Autodesk Fusion 360 part; units mm, degrees
(part 2 of 7)
sketch "Sketch32" plane through (0, 0, 15.6) normal (0, 0, 1) x (-1, 0, 0)
  circle A0 centre (0, 19.7) radius 11.5
  circle A1 centre (-93.9, 19.7) radius 11.5
  line L0 (-126.4, -25.2) -> (-93.9, -25.2)
  line L1 (-93.9, -25.2) -> (-93.9, 4.1)
  line L2 (-93.9, 4.1) -> (0, 4.1)
  line L3 (0, 4.1) -> (0, -25.2)
  line L4 (0, -25.2) -> (32.5, -25.2)
  line L5 (32.5, -25.2) -> (32.5, 25.3)
  arc A2 (32.5, 25.3) -> (22.5, 35.3) centre (22.5, 25.3) ccw
  line L6 (22.5, 35.3) -> (-110.15, 35.3)
  line L7 (-110.15, 35.3) -> (-116.4, 35.3)
  arc A3 (-116.4, 35.3) -> (-126.4, 25.3) centre (-116.4, 25.3) ccw
  line L8 (-126.4, 25.3) -> (-126.4, -25.2)
  line L9 (-66.7, 10) -> (-66.7, 30.4)
  line L10 (-27.2, 30.4) -> (-27.2, 10)
  line L11 (-29.2, 8) -> (-64.7, 8)
  line L12 (-27.2, 30.4) -> (-34.2, 30.4)
  line L13 (-34.2, 30.4) -> (-34.2, 32.4)
  line L14 (-59.7, 32.4) -> (-59.7, 30.4)
  line L15 (-59.7, 30.4) -> (-66.7, 30.4)
  arc A4 (-66.7, 10) -> (-64.7, 8) centre (-64.7, 10) ccw
  arc A5 (-29.2, 8) -> (-27.2, 10) centre (-29.2, 10) ccw
  line L16 (-34.2, 30.4) -> (-34.2, 32.4)
  line L17 (-34.2, 32.4) -> (-59.7, 32.4)
  point P0 (-27.2, 4.5)
  point P1 (-66.7, 33.9)
  dimension "d199" = 3.5
  dimension "d205" = 2
  constraint vertical L9
  constraint vertical L10
  constraint perpendicular L9 L11
  constraint perpendicular L12 L13
  constraint perpendicular L9 L15
  constraint perpendicular L12 L16
  constraint perpendicular L14 L17
  measures "d199" distance of P1 L9.end
  measures "d205" distance of L12.end L13.end
extrude "Extrude23" cut sketch "Sketch32" against normal blind 1 contours L9 L10 L11 L12 L13 L14 L15 A4 A5 L16 L17 bodies 6 7
sketch "Sketch34" plane through (0, 0, 15.6) normal (0, 0, 1) x (-1, 0, 0)
  line L0 (-34.2, 32.4) -> (-34.2, 30.4)
  line L1 (-34.2, 30.4) -> (-27.2, 30.4)
  line L2 (-27.2, 30.4) -> (-27.2, 10)
  arc A0 (-29.2, 8) -> (-27.2, 10) centre (-29.2, 10) ccw
  line L3 (-29.2, 8) -> (-64.7, 8)
  arc A1 (-66.7, 10) -> (-64.7, 8) centre (-64.7, 10) ccw
  line L4 (-66.7, 10) -> (-66.7, 30.4)
  line L5 (-66.7, 30.4) -> (-59.7, 30.4)
  line L6 (-59.7, 30.4) -> (-59.7, 32.4)
  line L7 (-59.7, 32.4) -> (-34.2, 32.4)
  line L8 (-126.4, -25.2) -> (-93.9, -25.2)
  line L9 (-93.9, -25.2) -> (-93.9, 4.1)
  line L10 (-93.9, 4.1) -> (0, 4.1)
  line L11 (0, 4.1) -> (0, -25.2)
  line L12 (0, -25.2) -> (32.5, -25.2)
  line L13 (32.5, -25.2) -> (32.5, 25.3)
  arc A2 (32.5, 25.3) -> (22.5, 35.3) centre (22.5, 25.3) ccw
  line L14 (22.5, 35.3) -> (-110.15, 35.3)
  line L15 (-110.15, 35.3) -> (-116.4, 35.3)
  arc A3 (-116.4, 35.3) -> (-126.4, 25.3) centre (-116.4, 25.3) ccw
  line L16 (-126.4, 25.3) -> (-126.4, -25.2)
  line L17 (-46.95, 4.1) -> (-46.95, -15) construction
  circle A4 centre (0, 19.7) radius 11.5
  circle A5 centre (0, 19.7) radius 11.5
  line L18 (9, 20.7) -> (-9, 20.7)
  line L19 (0, 10.7) -> (5, 10.7)
  line L20 (5, 10.7) -> (-5, 10.7)
  arc A6 (5, 10.7) -> (4.9996, 12.7) centre (5, 11.7) ccw
  arc A7 (-4.9996, 12.7) -> (-5, 10.7) centre (-5, 11.7) ccw
  line L21 (0, 12.7) -> (5.0004, 12.7)
  line L22 (5.0004, 12.7) -> (-5.0004, 12.7)
  line L23 (8.1652, 14.7) -> (-8.1652, 14.7)
  line L24 (0, 14.7) -> (8.1652, 14.7)
  line L25 (0, 16.7) -> (8.1652, 16.7)
  line L26 (8.1652, 16.7) -> (-8.1652, 16.7)
  arc A8 (8.1652, 14.7) -> (8.1652, 16.7) centre (8.1652, 15.7) ccw
  arc A9 (-8.1652, 16.7) -> (-8.1652, 14.7) centre (-8.1652, 15.7) ccw
  arc A10 (-9, 20.7) -> (-9, 18.7) centre (-9, 19.7) ccw
  line L27 (-9, 18.7) -> (9, 18.7)
  arc A11 (9, 18.7) -> (9, 20.7) centre (9, 19.7) ccw
  line L28 (5, 28.7) -> (-5, 28.7)
  arc A12 (4.9996, 26.7) -> (5, 28.7) centre (5, 27.7) ccw
  line L29 (5.0004, 26.7) -> (-5.0004, 26.7)
  arc A13 (-5, 28.7) -> (-4.9996, 26.7) centre (-5, 27.7) ccw
  line L30 (8.1652, 24.7) -> (-8.1652, 24.7)
  arc A14 (-8.1652, 24.7) -> (-8.1652, 22.7) centre (-8.1652, 23.7) ccw
  arc A15 (8.1652, 22.7) -> (8.1652, 24.7) centre (8.1652, 23.7) ccw
  line L31 (8.1652, 22.7) -> (-8.1652, 22.7)
  arc A16 (-84.9, 18.7) -> (-84.9, 20.7) centre (-84.9, 19.7) ccw
  circle A17 centre (-93.9, 19.7) radius 11.5
  arc A18 (-102.9, 20.7) -> (-102.9, 18.7) centre (-102.9, 19.7) ccw
  circle A19 centre (-93.9, 19.7) radius 11.5
  line L32 (-102.0652, 14.7) -> (-85.7348, 14.7)
  line L33 (-93.9, 16.7) -> (-102.0652, 16.7)
  arc A20 (-102.0652, 24.7) -> (-102.0652, 22.7) centre (-102.0652, 23.7) ccw
  arc A21 (-88.9, 10.7) -> (-88.9004, 12.7) centre (-88.9, 11.7) ccw
  line L34 (-102.9, 20.7) -> (-84.9, 20.7)
  line L35 (-93.9, 14.7) -> (-102.0652, 14.7)
  line L36 (-102.0652, 24.7) -> (-85.7348, 24.7)
  arc A22 (-98.9, 28.7) -> (-98.8996, 26.7) centre (-98.9, 27.7) ccw
  line L37 (-98.9004, 12.7) -> (-88.8996, 12.7)
  line L38 (-93.9, 12.7) -> (-98.9004, 12.7)
  line L39 (-93.9, 10.7) -> (-98.9, 10.7)
  line L40 (-84.9, 18.7) -> (-102.9, 18.7)
  line L41 (-98.9, 28.7) -> (-88.9, 28.7)
  arc A23 (-98.8996, 12.7) -> (-98.9, 10.7) centre (-98.9, 11.7) ccw
  arc A24 (-88.9004, 26.7) -> (-88.9, 28.7) centre (-88.9, 27.7) ccw
  line L42 (-98.9004, 26.7) -> (-88.8996, 26.7)
  arc A25 (-85.7348, 14.7) -> (-85.7348, 16.7) centre (-85.7348, 15.7) ccw
  line L43 (-102.0652, 22.7) -> (-85.7348, 22.7)
  arc A26 (-102.0652, 16.7) -> (-102.0652, 14.7) centre (-102.0652, 15.7) ccw
  line L44 (-98.9, 10.7) -> (-88.9, 10.7)
  arc A27 (-85.7348, 22.7) -> (-85.7348, 24.7) centre (-85.7348, 23.7) ccw
  line L45 (-102.0652, 16.7) -> (-85.7348, 16.7)
  point P0 (-11.5, 19.7)
  point P1 (-82.4, 19.7)
  dimension "d328" = 2
  constraint midpoint L10 L17.start
  constraint perpendicular L10 L17
  constraint concentric A4 A5
  constraint coincident P0 A5
  constraint coincident A6.end L21
  constraint coincident A7 L22.end
  constraint coincident A6 L21.end
  constraint symmetric L17 A4 A17
  constraint symmetric L17 P0 P1
  constraint symmetric L17 A5 A19
  constraint symmetric L17 L25.start L33.start
  constraint symmetric L17 L24.start L35.start
  constraint symmetric L17 L21.start L38.start
  constraint symmetric L17 L19.start L39.start
  constraint symmetric L17 L19.end L39.end
  constraint symmetric L17 A6 A23
  constraint symmetric L17 A6.end A23.start
  constraint symmetric L17 L20.end A21.start
  constraint symmetric L17 A7.start A21.end
  constraint symmetric L17 A7 A21
  constraint symmetric L17 L22.end L37.end
  constraint symmetric L17 L21.end L37.start
  constraint symmetric L17 L25.end L33.end
  constraint symmetric L17 L23.start L32.start
  constraint symmetric L17 A8 A26
  constraint symmetric L17 L23.end L32.end
  constraint symmetric L17 A9 A25
  constraint symmetric L17 L26.end A25.end
  constraint symmetric L17 A10.end A16.start
  constraint symmetric L17 A10 A16
  constraint symmetric L17 L18.end A16.end
  constraint symmetric L17 L18.start A18.start
  constraint symmetric L17 L27.end A18.end
  constraint symmetric L17 A11 A18
  constraint symmetric L17 L28.start A22.start
  constraint symmetric L17 L28.end L41.end
  constraint symmetric L17 A12.start A22.end
  constraint symmetric L17 A12 A22
  constraint symmetric L17 L29.start L42.start
  constraint symmetric L17 L29.end L42.end
  constraint symmetric L17 A13.end A24.start
  constraint symmetric L17 A13 A24
  constraint symmetric L17 L30.start A20.start
  constraint symmetric L17 L30.end L36.end
  constraint symmetric L17 A14.end L43.end
  constraint symmetric L17 A14 A27
  constraint symmetric L17 A15.start A20.end
  constraint symmetric L17 A15 A20
  measures "d328" distance of L24.start L21.start
extrude "Extrude26" add sketch "Sketch34" against normal blind 1 contours A4 A5 | A17 A19 bodies 7
sketch "Sketch35" plane through (0, 0, 14.6) normal (0, 0, -1) x (1, 0, 0)
  line L0 (88.8996, 12.7) -> (98.8996, 12.7)
  arc A0 (98.9, 10.7) -> (98.8996, 12.7) centre (98.9, 11.7) ccw
  line L1 (98.9, 10.7) -> (88.9, 10.7)
  arc A1 (88.8996, 12.7) -> (88.9, 10.7) centre (88.9, 11.7) ccw
  line L2 (102.0652, 14.7) -> (85.7348, 14.7)
  arc A2 (85.7348, 16.7) -> (85.7348, 14.7) centre (85.7348, 15.7) ccw
  line L3 (85.7348, 16.7) -> (102.0652, 16.7)
  arc A3 (102.0652, 14.7) -> (102.0652, 16.7) centre (102.0652, 15.7) ccw
  arc A4 (102.0652, 22.7) -> (102.0652, 24.7) centre (102.0652, 23.7) ccw
  line L4 (102.0652, 22.7) -> (85.7348, 22.7)
  arc A5 (85.7348, 24.7) -> (85.7348, 22.7) centre (85.7348, 23.7) ccw
  line L5 (85.7348, 24.7) -> (102.0652, 24.7)
  arc A6 (98.9004, 26.7) -> (98.9, 28.7) centre (98.9, 27.7) ccw
  line L6 (98.9004, 26.7) -> (88.8996, 26.7)
  arc A7 (88.9, 28.7) -> (88.8996, 26.7) centre (88.9, 27.7) ccw
  line L7 (88.9, 28.7) -> (98.9, 28.7)
  arc A8 (102.9, 18.7) -> (102.9, 20.7) centre (102.9, 19.7) ccw
  line L8 (102.9, 18.7) -> (84.9, 18.7)
  arc A9 (84.9, 20.7) -> (84.9, 18.7) centre (84.9, 19.7) ccw
  line L9 (84.9, 20.7) -> (102.9, 20.7)
  line L10 (8.1652, 14.7) -> (-8.1652, 14.7)
  arc A10 (-8.1652, 16.7) -> (-8.1652, 14.7) centre (-8.1652, 15.7) ccw
  line L11 (-8.1652, 16.7) -> (8.1652, 16.7)
  arc A11 (8.1652, 14.7) -> (8.1652, 16.7) centre (8.1652, 15.7) ccw
  arc A12 (-9, 20.7) -> (-9, 18.7) centre (-9, 19.7) ccw
  line L12 (-9, 20.7) -> (9, 20.7)
  arc A13 (9, 18.7) -> (9, 20.7) centre (9, 19.7) ccw
  line L13 (9, 18.7) -> (-9, 18.7)
  line L14 (-8.1652, 24.7) -> (8.1652, 24.7)
  arc A14 (8.1652, 22.7) -> (8.1652, 24.7) centre (8.1652, 23.7) ccw
  line L15 (8.1652, 22.7) -> (-8.1652, 22.7)
  arc A15 (-8.1652, 24.7) -> (-8.1652, 22.7) centre (-8.1652, 23.7) ccw
  arc A16 (-5, 28.7) -> (-5.0004, 26.7) centre (-5, 27.7) ccw
  line L16 (-5, 28.7) -> (5, 28.7)
  arc A17 (4.9996, 26.7) -> (5, 28.7) centre (5, 27.7) ccw
  line L17 (4.9996, 26.7) -> (-5.0004, 26.7)
  arc A18 (-5.0004, 12.7) -> (-5, 10.7) centre (-5, 11.7) ccw
  line L18 (-5.0004, 12.7) -> (5.0004, 12.7)
  arc A19 (5, 10.7) -> (5.0004, 12.7) centre (5, 11.7) ccw
  line L19 (5, 10.7) -> (-5, 10.7)
  line L20 (34.2, 30.4) -> (34.2, 32.4)
  line L21 (34.2, 32.4) -> (59.7, 32.4)
  line L22 (59.7, 32.4) -> (59.7, 30.4)
  line L23 (59.7, 30.4) -> (66.7, 30.4)
  line L24 (66.7, 30.4) -> (66.7, 10)
  arc A20 (64.7, 8) -> (66.7, 10) centre (64.7, 10) ccw
  line L25 (64.7, 8) -> (29.2, 8)
  arc A21 (27.2, 10) -> (29.2, 8) centre (29.2, 10) ccw
  line L26 (27.2, 10) -> (27.2, 30.4)
  line L27 (27.2, 30.4) -> (34.2, 30.4)
  line L28 (93.9, -25.2) -> (126.4, -25.2)
  line L29 (126.4, -25.2) -> (126.4, 25.3)
  arc A22 (126.4, 25.3) -> (116.4, 35.3) centre (116.4, 25.3) ccw
  line L30 (116.4, 35.3) -> (110.15, 35.3)
  line L31 (110.15, 35.3) -> (-22.5, 35.3)
  arc A23 (-22.5, 35.3) -> (-32.5, 25.3) centre (-22.5, 25.3) ccw
  line L32 (-32.5, 25.3) -> (-32.5, -25.2)
  line L33 (-32.5, -25.2) -> (0, -25.2)
  line L34 (0, -25.2) -> (0, 4.1)
  line L35 (0, 4.1) -> (93.9, 4.1)
  line L36 (93.9, 4.1) -> (93.9, -25.2)
  circle A24 centre (0, 19.7) radius 11.5
  circle A25 centre (0, 19.7) radius 14
  line L37 (46.95, 4.1) -> (46.95, -7.4163) construction
  circle A26 centre (93.9, 19.7) radius 14
  circle A27 centre (93.9, 19.7) radius 11.5
  point P0 (0, 19.7)
  dimension "d335" = 28
  constraint coincident P0 A24.centre
  constraint midpoint L35 L37.start
  constraint perpendicular L35 L37
  constraint symmetric A24 L37 A27
  constraint symmetric A25 L37 A26
  measures "d335" diameter of A25
extrude "Extrude27" add sketch "Sketch35" along normal blind 1.5 contours A25 | A26 bodies 7
extrude "Extrude28" add 1 faces at (-10.2309, 68.7361, 13.1) along direction (0, 0, -1) blind 3.1 on bodies 5 bodies 5
sketch "Sketch36" plane through (0, 0, 10) normal (0, 0, -1) x (1, 0, 0)
  arc A0 (-32.5, -65.1) -> (-12.5, -85.1) centre (-12.5, -65.1) ccw
  line L0 (-12.5, -85.1) -> (106.4, -85.1)
  arc A1 (106.4, -85.1) -> (126.2303, -67.7) centre (106.4, -65.1) ccw
  line L1 (126.2303, -67.7) -> (93.9, -67.7)
  line L2 (93.9, -67.7) -> (93.9, -75.1)
  line L3 (93.9, -75.1) -> (0, -75.1)
  line L4 (0, -75.1) -> (0, -57.7)
  line L5 (0, -57.7) -> (-32.5, -57.7)
  line L6 (-32.5, -57.7) -> (-32.5, -65.1)
  line L7 (93.9, -75.1) -> (0, -75.1)
  line L8 (46.95, -75.1) -> (46.95, -85.1)
  line L9 (46.95, -80.1) -> (46.95, -77.15)
  circle A2 centre (46.95, -80.1) radius 2.95
  dimension "d340" = 2.95
  constraint coincident L2.end L3.start
  constraint coincident L3.end L4.start
  constraint midpoint L3 L8.start
  constraint midpoint L0 L8.end
  constraint midpoint L8 L9.start
  constraint perpendicular L0 L9
  constraint coincident L9.start A2.centre
  constraint coincident L9.end A2
  measures "d340" distance of L9.start L9.end
extrude "Extrude29" cut sketch "Sketch36" against normal blind 10 contours L8 L9 A2 | L8 L9 A2 bodies 5
sketch "Sketch37" plane through (0, 0, 15.6) normal (0, 0, 1) x (-1, 0, 0)
  circle A0 centre (-46.95, -80.1) radius 2.95
  arc A1 (12.5, -85.1) -> (32.5, -65.1) centre (12.5, -65.1) ccw
  line L0 (32.5, -65.1) -> (32.5, -57.7)
  line L1 (32.5, -57.7) -> (0, -57.7)
  line L2 (0, -57.7) -> (0, -75.1)
  line L3 (0, -75.1) -> (-93.9, -75.1)
  line L4 (-93.9, -75.1) -> (-93.9, -67.7)
  line L5 (-93.9, -67.7) -> (-126.2303, -67.7)
  arc A2 (-126.2303, -67.7) -> (-106.4, -85.1) centre (-106.4, -65.1) ccw
  line L6 (-106.4, -85.1) -> (12.5, -85.1)
  circle A3 centre (-46.95, -80.1) radius 2.95
  arc A4 (-47.45, -80.6) -> (-46.45, -80.6) centre (-46.95, -80.6) ccw
  arc A5 (-46.45, -79.6) -> (-47.45, -79.6) centre (-46.95, -79.6) ccw
  arc A6 (-45.65, -80.6) -> (-45.65, -79.6) centre (-45.65, -80.1) ccw
  line L7 (-45.65, -80.6) -> (-46.45, -80.6)
  line L8 (-47.45, -80.6) -> (-48.25, -80.6)
  line L9 (-48.25, -79.6) -> (-47.45, -79.6)
  line L10 (-46.45, -79.6) -> (-45.65, -79.6)
  arc A7 (-48.25, -79.6) -> (-48.25, -80.6) centre (-48.25, -80.1) ccw
  line L11 (-46.45, -80.6) -> (-47.45, -80.6)
  constraint concentric A0 A3
  constraint collinear L7 L8
  constraint collinear L9 L10
extrude "Extrude31" add sketch "Sketch37" against normal blind 1 contours A0 A3 bodies 5
sketch "Sketch39" plane through (0, 0, 14.6) normal (0, 0, -1) x (1, 0, 0)
  circle A0 centre (0, 19.7) radius 14
  line L0 (34.2, 30.4) -> (34.2, 32.4)
  line L1 (34.2, 32.4) -> (59.7, 32.4)
  line L2 (59.7, 32.4) -> (59.7, 30.4)
  line L3 (59.7, 30.4) -> (66.7, 30.4)
  line L4 (66.7, 30.4) -> (66.7, 10)
  arc A1 (64.7, 8) -> (66.7, 10) centre (64.7, 10) ccw
  line L5 (64.7, 8) -> (29.2, 8)
  arc A2 (27.2, 10) -> (29.2, 8) centre (29.2, 10) ccw
  line L6 (27.2, 10) -> (27.2, 30.4)
  line L7 (27.2, 30.4) -> (34.2, 30.4)
  line L8 (93.9, -25.2) -> (126.4, -25.2)
  line L9 (126.4, -25.2) -> (126.4, 25.3)
  arc A3 (126.4, 25.3) -> (116.4, 35.3) centre (116.4, 25.3) ccw
  line L10 (116.4, 35.3) -> (110.15, 35.3)
  line L11 (110.15, 35.3) -> (-22.5, 35.3)
  arc A4 (-22.5, 35.3) -> (-32.5, 25.3) centre (-22.5, 25.3) ccw
  line L12 (-32.5, 25.3) -> (-32.5, -25.2)
  line L13 (-32.5, -25.2) -> (0, -25.2)
  line L14 (0, -25.2) -> (0, 4.1)
  line L15 (0, 4.1) -> (93.9, 4.1)
  line L16 (93.9, 4.1) -> (93.9, -25.2)
  circle A5 centre (93.9, 19.7) radius 14
  line L17 (66.7, 4.5) -> (66.7, 4.1)
  line L18 (66.7, 4.1) -> (93.9, 4.1)
  line L19 (93.9, 4.1) -> (126.4, 4.1)
  line L20 (126.4, 4.1) -> (126.4, 25.3)
  line L21 (116.4, 35.3) -> (-22.5, 35.3)
  arc A6 (126.4, 25.3) -> (116.4, 35.3) centre (116.4, 25.3) ccw
  circle A7 centre (93.9, 19.7) radius 14
  line L22 (66.7, 4.5) -> (66.7, 33.9)
  line L23 (66.7, 33.9) -> (27.2, 33.9)
  line L24 (27.2, 33.9) -> (27.2, 4.1)
  line L25 (27.2, 4.1) -> (0, 4.1)
  line L26 (0, 4.1) -> (-32.5, 4.1)
  line L27 (-32.5, 4.1) -> (-32.5, 25.3)
  arc A8 (-22.5, 35.3) -> (-32.5, 25.3) centre (-22.5, 25.3) ccw
  circle A9 centre (0, 19.7) radius 14
  point P0 (66.7, 4.5)
  point P1 (79.9, 19.7)
  point P2 (66.7, 33.9)
  point P3 (27.2, 33.9)
  point P4 (-14, 19.7)
  constraint coincident P0 L17.start
  constraint coincident L15 L17.end
  constraint perpendicular L15 L17
  constraint coincident L15.end L16.start
  constraint coincident L9 L19.end
  constraint perpendicular L9 L19
  constraint coincident L9.end A3.start
  constraint coincident A3.end L10.start
  constraint coincident L11.end A4.start
  constraint concentric A5 A7
  constraint coincident A7 P1
  constraint coincident P2 L22.end
  constraint coincident P3 L23.end
  constraint coincident L15 L24.end
  constraint perpendicular L15 L24
  constraint coincident L14.end L15.start
  constraint coincident L12 L26.end
  constraint perpendicular L12 L26
  constraint coincident A4.end L12.start
  constraint coincident A4.end A8
  constraint concentric A0 A9
  constraint coincident A9 P4
extrude "Extrude32" add sketch "Sketch39" along normal blind 4.6 contours L4 L6 L9 A3 L10 L11 A4 L12 L15 L17 L18 L19 L20 L21 A6 L22 L23 L24 L25 L26 L27 A8 bodies 7
sketch "Sketch40" plane through (66.7, 0, 0) normal (-1, 0, 0) x (0, -1, 0)
  line L0 (30.4, 15.6) -> (10, 15.6)
  line L1 (10, 15.6) -> (10, 14.6)
  line L2 (10, 14.6) -> (4.1, 14.6)
  line L3 (4.1, 14.6) -> (4.1, 10)
  line L4 (4.1, 10) -> (33.9, 10)
  line L5 (33.9, 10) -> (33.9, 14.6)
  line L6 (33.9, 14.6) -> (30.4, 14.6)
  line L7 (30.4, 14.6) -> (30.4, 15.6)
  line L8 (4.1, 14.6) -> (8.7, 10)
  line L9 (4.1, 14.6) -> (10.6054, 14.6) construction
  line L10 (8.7, 10) -> (4.1, 10)
  line L11 (4.1, 14.6) -> (4.1, 10)
  dimension "d363" = 45
  constraint horizontal L9
  constraint coincident L2.end L3.start
  constraint coincident L4 L8.end
  constraint coincident L3.end L4.start
  measures "d363" angle of L8 L9
extrude "Extrude33" cut sketch "Sketch40" against normal blind 27.2 contours L3 L4 L8 L10 L11 bodies 7
sketch "Sketch42" plane through (27.2, 0, 0) normal (1, 0, 0) x (0, 1, 0)
  line L0 (-10, 15.6) -> (-30.4, 15.6)
  line L1 (-30.4, 15.6) -> (-30.4, 14.6)
  line L2 (-30.4, 14.6) -> (-33.9, 14.6)
  line L3 (-33.9, 14.6) -> (-33.9, 10)
  line L4 (-33.9, 10) -> (-4.1, 10)
  line L5 (-4.1, 10) -> (-4.1, 14.6)
  line L6 (-4.1, 14.6) -> (-10, 14.6)
  line L7 (-10, 14.6) -> (-10, 15.6)
  line L8 (-4.1, 14.6) -> (-8.7, 10)
  line L9 (-4.1, 14.6) -> (2.4054, 14.6) construction
  line L10 (-8.7, 10) -> (-4.1, 10)
  line L11 (-4.1, 10) -> (-4.1, 14.6)
  dimension "d369" = 135
  constraint horizontal L9
  constraint coincident L5.end L6.start
  constraint coincident L4 L8.end
  constraint coincident L4.end L5.start
  measures "d369" angle of L8 L9
extrude "Extrude35" cut sketch "Sketch42" against normal blind 27.2 contours L4 L5 L8 L10 L11 bodies 7
sketch "Sketch43" plane through (0, 0, 14.6) normal (0, 0, -1) x (1, 0, 0)
  line L0 (126.4, 4.1) -> (93.9, 4.1)
  line L1 (93.9, 4.1) -> (93.9, -25.2)
  line L2 (93.9, -25.2) -> (126.4, -25.2)
  line L3 (126.4, -25.2) -> (126.4, 4.1)
  line L4 (93.9, -25.2) -> (95.9, -25.2)
  line L5 (93.9, 4.1) -> (95.9, 4.1)
  line L6 (126.2303, -67.7) -> (93.9, -67.7)
  line L7 (93.9, -67.7) -> (95.9, -67.7)
  line L8 (95.9, -67.7) -> (95.9, 4.1)
  line L9 (93.9, 4.1) -> (93.9, -67.7)
  line L10 (0, -57.7) -> (-2, -57.7)
  line L11 (-32.5, 4.1) -> (0, 4.1)
  line L12 (0, 4.1) -> (-2, 4.1)
  line L13 (-2, -57.7) -> (-2, 4.1)
  line L14 (0, 4.1) -> (0, -57.7)
  point P0 (93.9, -67.7)
  point P1 (0, -57.7)
  point P2 (0, 4.1)
  dimension "d372" = 2
  dimension "d373" = 2
  dimension "d374" = 2
  dimension "d375" = 2
  dimension "d376" = 2
  constraint coincident L1.end L2.start
  constraint perpendicular L1 L4
  constraint coincident L0.end L1.start
  constraint perpendicular L1 L5
  constraint coincident P0 L6.end
  constraint parallel L6 L7
  constraint coincident P1 L10.start
  constraint perpendicular L9 L10
  constraint coincident P2 L11.end
  constraint parallel L11 L12
  measures "d372" distance of L1.end L4.end
  measures "d373" distance of L0.end L5.end
  measures "d374" distance of P0 L7.end
  measures "d375" distance of P1 L10.end
  measures "d376" distance of P2 L12.end
extrude "Extrude36" add sketch "Sketch43" along normal blind 4.6 contours L0 L1 L2 L4 L5 L8 L9 | L2 L4 L6 L7 L8 L9 | L10 L11 L12 L13 L14 bodies 3 4 5 7
sketch "Sketch44" plane through (0, 0, 10) normal (0, 0, -1) x (1, 0, 0)
  line L0 (-2, -57.7) -> (-32.5, -57.7)
  line L1 (-32.5, -57.7) -> (-32.5, -65.1)
  arc A0 (-32.5, -65.1) -> (-12.5, -85.1) centre (-12.5, -65.1) ccw
  line L2 (-12.5, -85.1) -> (106.4, -85.1)
  arc A1 (106.4, -85.1) -> (126.2303, -67.7) centre (106.4, -65.1) ccw
  line L3 (126.2303, -67.7) -> (95.9, -67.7)
  line L4 (95.9, -67.7) -> (95.9, 4.1)
  line L5 (95.9, 4.1) -> (126.4, 4.1)
  line L6 (126.4, 4.1) -> (126.4, 25.3)
  arc A2 (126.4, 25.3) -> (116.4, 35.3) centre (116.4, 25.3) ccw
  line L7 (116.4, 35.3) -> (-22.5, 35.3)
  arc A3 (-22.5, 35.3) -> (-32.5, 25.3) centre (-22.5, 25.3) ccw
  line L8 (-32.5, 25.3) -> (-32.5, 4.1)
  line L9 (-32.5, 4.1) -> (-2, 4.1)
  line L10 (-2, 4.1) -> (-2, -57.7)
  circle A4 centre (46.95, -80.1) radius 2.95
  line L11 (0, -75.1) -> (0, 5.7)
  arc A5 (8.6603, 8.7) -> (0, 5.7) centre (0, 19.7) ccw
  line L12 (8.6603, 8.7) -> (27.2, 8.7)
  line L13 (27.2, 8.7) -> (27.2, 33.9)
  line L14 (27.2, 33.9) -> (66.7, 33.9)
  line L15 (66.7, 33.9) -> (66.7, 8.7)
  line L16 (66.7, 8.7) -> (85.2397, 8.7)
  arc A6 (93.9, 5.7) -> (85.2397, 8.7) centre (93.9, 19.7) ccw
  line L17 (93.9, 5.7) -> (93.9, -75.1)
  line L18 (93.9, -75.1) -> (0, -75.1)
  line L19 (95.9, -67.7) -> (129, -67.7)
  line L20 (129, -67.7) -> (129, -88)
  line L21 (129, -88) -> (95.9, -88)
  line L22 (95.9, -88) -> (95.9, -67.7)
  line L23 (-2, -57.7) -> (-36.3118, -57.7)
  line L24 (-36.3118, -57.7) -> (-36.3118, -88)
  line L25 (-36.3118, -88) -> (-2, -88)
  line L26 (-2, -88) -> (-2, -57.7)
  constraint horizontal L19
  constraint vertical L20
  constraint horizontal L21
  constraint vertical L22
  constraint coincident L3.end L4.start
  constraint horizontal L23
  constraint vertical L24
  constraint horizontal L25
  constraint vertical L26
  constraint coincident L0.start L10.end
extrude "Extrude37" cut sketch "Sketch44" against normal blind 4.6 contours L0 L1 A0 L2 L23 L26 | L2 A1 L3 L19 L22 bodies 3
sketch "Sketch45" plane through (0, 0, 10) normal (0, 0, -1) x (1, 0, 0)
  line L0 (0, -75.1) -> (0, 5.7)
  arc A0 (8.6603, 8.7) -> (0, 5.7) centre (0, 19.7) ccw
  line L1 (8.6603, 8.7) -> (27.2, 8.7)
  line L2 (27.2, 8.7) -> (27.2, 33.9)
  line L3 (27.2, 33.9) -> (66.7, 33.9)
  line L4 (66.7, 33.9) -> (66.7, 8.7)
  line L5 (66.7, 8.7) -> (85.2397, 8.7)
  arc A1 (93.9, 5.7) -> (85.2397, 8.7) centre (93.9, 19.7) ccw
  line L6 (93.9, 5.7) -> (93.9, -75.1)
  line L7 (93.9, -75.1) -> (0, -75.1)
  circle A2 centre (46.95, -80.1) radius 2.95
  line L8 (95.9, -85.1) -> (95.9, 4.1)
  line L9 (95.9, 4.1) -> (126.4, 4.1)
  line L10 (126.4, 4.1) -> (126.4, 25.3)
  arc A3 (126.4, 25.3) -> (116.4, 35.3) centre (116.4, 25.3) ccw
  line L11 (116.4, 35.3) -> (-22.5, 35.3)
  arc A4 (-22.5, 35.3) -> (-32.5, 25.3) centre (-22.5, 25.3) ccw
  line L12 (-32.5, 25.3) -> (-32.5, 4.1)
  line L13 (-32.5, 4.1) -> (-2, 4.1)
  line L14 (-2, 4.1) -> (-2, -85.1)
  line L15 (-2, -85.1) -> (95.9, -85.1)
  line L16 (93.9, -75.1) -> (93.9, -77.2)
  line L17 (93.9, -77.2) -> (95.9, -77.2)
  line L18 (95.9, -77.2) -> (75.9, -77.2)
  line L19 (75.9, -77.2) -> (95.9, -77.2)
  line L20 (95.9, -77.2) -> (95.9, -85.1)
  line L21 (95.9, -85.1) -> (75.9, -85.1)
  line L22 (75.9, -85.1) -> (75.9, -77.2)
  dimension "d381" = 2.1
  dimension "d382" = 20
  constraint coincident L6.end L7.start
  constraint perpendicular L7 L16
  constraint coincident L8 L17.end
  constraint perpendicular L8 L17
  constraint perpendicular L8 L18
  constraint horizontal L19
  constraint vertical L20
  constraint horizontal L21
  constraint vertical L22
  constraint coincident L8.start L15.end
  measures "d381" distance of L6.end L16.end
  measures "d382" distance of L17.end L18.end
extrude "Extrude38" cut sketch "Sketch45" against normal blind 4.6 contours L8 L15 L17 L18 L19 L20 L21 L22 bodies 3
sketch "Sketch46" plane through (0, 0, 14.6) normal (0, 0, -1) x (1, 0, 0)
  line L0 (95.9, 4.1) -> (95.9, -77.2)
  line L1 (95.9, -77.2) -> (75.9, -77.2)
  line L2 (75.9, -77.2) -> (75.9, -85.1)
  line L3 (75.9, -85.1) -> (106.4, -85.1)
  arc A0 (106.4, -85.1) -> (126.4, -65.1) centre (106.4, -65.1) ccw
  line L4 (126.4, -65.1) -> (126.4, 4.1)
  line L5 (126.4, 4.1) -> (95.9, 4.1)
  line L6 (107.5299, -38.2671) -> (107.1448, -38.6523)
  line L7 (107.1448, -38.6523) -> (105.4477, -36.9552)
  line L8 (105.4477, -36.9552) -> (105.8329, -36.5701)
  arc A1 (107.9591, -29.4) -> (105.8329, -36.5701) centre (110.15, -33.95) ccw
  line L9 (107.9591, -29.4) -> (112.3409, -29.4)
  arc A2 (112.3409, -38.5) -> (112.3409, -29.4) centre (110.15, -33.95) ccw
  line L10 (112.3409, -38.5) -> (107.9591, -38.5)
  arc A3 (107.5299, -38.2671) -> (107.9591, -38.5) centre (110.15, -33.95) ccw
  line L11 (112.7701, -44.6329) -> (113.1552, -44.2477)
  line L12 (113.1552, -44.2477) -> (114.8523, -45.9448)
  line L13 (114.8523, -45.9448) -> (114.4671, -46.3299)
  arc A4 (112.3364, -53.5022) -> (114.4671, -46.3299) centre (110.15, -48.95) ccw
  line L14 (112.3364, -53.5022) -> (112.3364, -53.5)
  line L15 (112.3364, -53.5) -> (107.9591, -53.5)
  arc A5 (107.9591, -44.4) -> (107.9591, -53.5) centre (110.15, -48.95) ccw
  line L16 (107.9591, -44.4) -> (112.3409, -44.4)
  arc A6 (112.7701, -44.6329) -> (112.3409, -44.4) centre (110.15, -48.95) ccw
  line L17 (106.9671, -44.0701) -> (107.3523, -44.4552)
  line L18 (107.3523, -44.4552) -> (105.6552, -46.1523)
  line L19 (105.6552, -46.1523) -> (105.2701, -45.7671)
  arc A7 (98.115, -43.6717) -> (105.2701, -45.7671) centre (102.65, -41.45) ccw
  line L20 (98.115, -43.6717) -> (98.0852, -39.29)
  arc A8 (107.185, -39.2283) -> (98.0852, -39.29) centre (102.65, -41.45) ccw
  line L21 (107.185, -39.2283) -> (107.2148, -43.61)
  arc A9 (106.9671, -44.0701) -> (107.2148, -43.61) centre (102.65, -41.45) ccw
  line L22 (113.3329, -38.8299) -> (112.9477, -38.4448)
  line L23 (112.9477, -38.4448) -> (114.6448, -36.7477)
  line L24 (114.6448, -36.7477) -> (115.0299, -37.1329)
  arc A10 (122.2, -39.2591) -> (115.0299, -37.1329) centre (117.65, -41.45) ccw
  line L25 (122.2, -39.2591) -> (122.2, -43.6409)
  arc A11 (113.1, -43.6409) -> (122.2, -43.6409) centre (117.65, -41.45) ccw
  line L26 (113.1, -43.6409) -> (113.1, -39.2591)
  arc A12 (113.3329, -38.8299) -> (113.1, -39.2591) centre (117.65, -41.45) ccw
  circle A13 centre (102.6547, -56.4453) radius 2.85
  circle A14 centre (117.6453, -56.4453) radius 2.85
  line L27 (93.9, -75.1) -> (93.9, -62.1)
  line L28 (110.15, -48.95) -> (110.15, -75) construction
  line L29 (93.9, -62.1) -> (111.5, -62.1)
  line L30 (110.15, -62.1) -> (107.65, -62.1)
  circle A15 centre (110.15, -62.1) radius 2.5
  line L31 (126.4, -65.1) -> (-32.5, -65.1)
  line L32 (93.9, -62.1) -> (93.9, -65.1)
  line L33 (-2, -65.1) -> (-2, -62.1)
  line L34 (-2, -62.1) -> (-16.25, -62.1)
  circle A16 centre (-16.25, -62.1) radius 2.5
  line L35 (102.65, -41.45) -> (87.8982, -41.4191) construction
  circle A17 centre (110.2363, -20.8316) radius 2.5
  circle A18 centre (-16.1626, -20.3028) radius 2.5
  point P0 (93.9, -75.1)
  point P1 (-32.5, -65.1)
  dimension "d385" = 13
  dimension "d386" = 2.5
  dimension "d387" = 3
  dimension "d388" = 14.25
  dimension "d389" = 5
  constraint coincident P0 L27.start
  constraint parallel L0 L27
  constraint coincident A4.centre A5.centre
  constraint perpendicular L15 L28
  constraint perpendicular L28 L29
  constraint coincident L29 L30.start
  constraint coincident L28 L30.start
  constraint perpendicular L28 L30
  constraint coincident L30.start A15.centre
  constraint coincident L30.end A15
  constraint coincident A0.end L4.start
  constraint coincident P1 L31.end
  constraint coincident L27 L32.end
  constraint coincident L31 L32.end
  constraint coincident L31 L33.start
  constraint perpendicular L31 L33
  constraint perpendicular L33 L34
  constraint coincident L34.end A16.centre
  constraint coincident A7.centre A8.centre
  constraint symmetric A15 L35 A17
  constraint symmetric A16 L35 A18
  measures "d385" distance of P0 L27.end
  measures "d386" distance of L30.start L30.end
  measures "d387" distance of L33.start L33.end
  measures "d388" distance of L33.end L34.end
  measures "d389" diameter of A16
extrude "Extrude39" add sketch "Sketch46" along normal blind 1.6 contours A15 | A16 bodies 3
extrude "Extrude40" add sketch "Sketch46" along normal blind 1.6 contours A15 | A16 | A17 | A18 bodies 3
sketch "Sketch48" plane through (0, 0, 13) normal (0, 0, -1) x (1, 0, 0)
  circle A0 centre (110.15, -62.1) radius 2.5
  line L0 (110.15, -62.1) -> (109.75, -62.1)
  circle A1 centre (110.15, -62.1) radius 0.4
  circle A2 centre (110.2363, -20.8316) radius 0.4
  circle A3 centre (110.2363, -20.8316) radius 2.5
  circle A4 centre (-16.25, -62.1) radius 0.4
  circle A5 centre (-16.25, -62.1) radius 2.5
  circle A6 centre (-16.1626, -20.3028) radius 0.4
  circle A7 centre (-16.1626, -20.3028) radius 2.5
  dimension "d400" = 0.4
  dimension "d401" = 0.8
  dimension "d402" = 0.8
  dimension "d403" = 0.8
  constraint coincident A0.centre L0.start
  constraint horizontal L0
  constraint coincident L0.end A1
  constraint concentric A2 A3
  constraint concentric A4 A5
  constraint concentric A6 A7
  measures "d400" distance of A0.centre L0.end
  measures "d401" diameter of A2
  measures "d402" diameter of A4
  measures "d403" diameter of A6
extrude "Extrude42" cut sketch "Sketch48" against normal blind 0.5 contours A1 | A2 | A4 | A6 bodies 3
sketch "Sketch49" plane through (0, 0, 10) normal (0, 0, -1) x (1, 0, 0)
  line L0 (75.9, -77.2) -> (95.9, -77.2)
  line L1 (95.9, -77.2) -> (95.9, 4.1)
  line L2 (95.9, 4.1) -> (126.4, 4.1)
  line L3 (126.4, 4.1) -> (126.4, 25.3)
  arc A0 (126.4, 25.3) -> (116.4, 35.3) centre (116.4, 25.3) ccw
  line L4 (116.4, 35.3) -> (-22.5, 35.3)
  arc A1 (-22.5, 35.3) -> (-32.5, 25.3) centre (-22.5, 25.3) ccw
  line L5 (-32.5, 25.3) -> (-32.5, 4.1)
  line L6 (-32.5, 4.1) -> (-2, 4.1)
  line L7 (-2, 4.1) -> (-2, -85.1)
  line L8 (-2, -85.1) -> (75.9, -85.1)
  line L9 (75.9, -85.1) -> (75.9, -77.2)
  line L10 (0, -75.1) -> (0, 5.7)
  arc A2 (8.6603, 8.7) -> (0, 5.7) centre (0, 19.7) ccw
  line L11 (8.6603, 8.7) -> (27.2, 8.7)
  line L12 (27.2, 8.7) -> (27.2, 33.9)
  line L13 (27.2, 33.9) -> (66.7, 33.9)
  line L14 (66.7, 33.9) -> (66.7, 8.7)
  line L15 (66.7, 8.7) -> (85.2397, 8.7)
  arc A3 (93.9, 5.7) -> (85.2397, 8.7) centre (93.9, 19.7) ccw
  line L16 (93.9, 5.7) -> (93.9, -75.1)
  line L17 (93.9, -75.1) -> (0, -75.1)
  circle A4 centre (46.95, -80.1) radius 2.95
  line L18 (95.9, -77.2) -> (-2, -77.2)
  line L19 (-2, -77.2) -> (-2, 4.1)
  line L20 (-2, 4.1) -> (95.9, 4.1)
  line L21 (95.9, 4.1) -> (95.9, -77.2)
  line L22 (93.9, -75.1) -> (0, -75.1)
  line L23 (0, -75.1) -> (0, 4.1)
  line L24 (0, 4.1) -> (93.9, 4.1)
  line L25 (93.9, 4.1) -> (93.9, -75.1)
  point P0 (0, 4.1)
  constraint horizontal L18
  constraint vertical L19
  constraint horizontal L20
  constraint vertical L21
  constraint coincident L6.end L7.start
  constraint coincident L0.end L1.start
  constraint horizontal L22
  constraint vertical L23
  constraint horizontal L24
  constraint vertical L25
  constraint coincident P0 L23.end
  constraint coincident L16.end L17.start
extrude "Extrude43" add sketch "Sketch49" along normal blind 6 contours L0 L1 L7 L10 L16 L17 A4 L18 L19 L20 L21 L22 L23 L25 bodies 3
sketch "Sketch52" plane through (0, 0, 14.6) normal (0, 0, -1) x (1, 0, 0)
  circle A0 centre (110.2363, -20.8316) radius 2.5
  circle A1 centre (110.15, -62.1) radius 2.5
  line L0 (95.9, 4.1) -> (95.9, -77.2)
  line L1 (95.9, -77.2) -> (75.9, -77.2)
  line L2 (75.9, -77.2) -> (75.9, -85.1)
  line L3 (75.9, -85.1) -> (106.4, -85.1)
  arc A2 (106.4, -85.1) -> (126.4, -65.1) centre (106.4, -65.1) ccw
  line L4 (126.4, -65.1) -> (126.4, 4.1)
  line L5 (126.4, 4.1) -> (95.9, 4.1)
  line L6 (107.5299, -38.2671) -> (107.1448, -38.6523)
  line L7 (107.1448, -38.6523) -> (105.4477, -36.9552)
  line L8 (105.4477, -36.9552) -> (105.8329, -36.5701)
  arc A3 (107.9591, -29.4) -> (105.8329, -36.5701) centre (110.15, -33.95) ccw
  line L9 (107.9591, -29.4) -> (112.3409, -29.4)
  arc A4 (112.3409, -38.5) -> (112.3409, -29.4) centre (110.15, -33.95) ccw
  line L10 (112.3409, -38.5) -> (107.9591, -38.5)
  arc A5 (107.5299, -38.2671) -> (107.9591, -38.5) centre (110.15, -33.95) ccw
  line L11 (112.7701, -44.6329) -> (113.1552, -44.2477)
  line L12 (113.1552, -44.2477) -> (114.8523, -45.9448)
  line L13 (114.8523, -45.9448) -> (114.4671, -46.3299)
  arc A6 (112.3364, -53.5022) -> (114.4671, -46.3299) centre (110.15, -48.95) ccw
  line L14 (112.3364, -53.5022) -> (112.3364, -53.5)
  line L15 (112.3364, -53.5) -> (107.9591, -53.5)
  arc A7 (107.9591, -44.4) -> (107.9591, -53.5) centre (110.15, -48.95) ccw
  line L16 (107.9591, -44.4) -> (112.3409, -44.4)
  arc A8 (112.7701, -44.6329) -> (112.3409, -44.4) centre (110.15, -48.95) ccw
  line L17 (106.9671, -44.0701) -> (107.3523, -44.4552)
  line L18 (107.3523, -44.4552) -> (105.6552, -46.1523)
  line L19 (105.6552, -46.1523) -> (105.2701, -45.7671)
  arc A9 (98.115, -43.6717) -> (105.2701, -45.7671) centre (102.65, -41.45) ccw
  line L20 (98.115, -43.6717) -> (98.0852, -39.29)
  arc A10 (107.185, -39.2283) -> (98.0852, -39.29) centre (102.65, -41.45) ccw
  line L21 (107.185, -39.2283) -> (107.2148, -43.61)
  arc A11 (106.9671, -44.0701) -> (107.2148, -43.61) centre (102.65, -41.45) ccw
  line L22 (113.3329, -38.8299) -> (112.9477, -38.4448)
  line L23 (112.9477, -38.4448) -> (114.6448, -36.7477)
  line L24 (114.6448, -36.7477) -> (115.0299, -37.1329)
  arc A12 (122.2, -39.2591) -> (115.0299, -37.1329) centre (117.65, -41.45) ccw
  line L25 (122.2, -39.2591) -> (122.2, -43.6409)
  arc A13 (113.1, -43.6409) -> (122.2, -43.6409) centre (117.65, -41.45) ccw
  line L26 (113.1, -43.6409) -> (113.1, -39.2591)
  arc A14 (113.3329, -38.8299) -> (113.1, -39.2591) centre (117.65, -41.45) ccw
  circle A15 centre (102.6547, -56.4453) radius 2.85
  circle A16 centre (117.6453, -56.4453) radius 2.85
  line L27 (95.9, 4.1) -> (95.9, -0.9)
  line L28 (95.9, -0.9) -> (98.4, -0.9)
  line L29 (95.9, 4.1) -> (98.4, 4.1)
  line L30 (100.9, 1.6) -> (100.9, 4.1)
  line L31 (100.9, 4.1) -> (95.9, 4.1)
  circle A17 centre (98.4, 1.6) radius 0.4
  line L32 (93.9, -75.1) -> (0, -75.1)
  line L33 (46.95, -75.1) -> (46.95, -46.628) construction
  circle A18 centre (-4.5, 1.6) radius 0.4
  line L34 (-2, -0.9) -> (-4.5, -0.9)
  line L35 (-7, 1.6) -> (-7, 4.1)
  line L36 (-2, 4.1) -> (-4.5, 4.1)
  line L37 (-2, 4.1) -> (-2, 1.6)
  arc A19 (-7, 1.6) -> (-4.5, -0.9) centre (-4.5, 1.6) ccw
  arc A20 (98.4, -0.9) -> (100.9, 1.6) centre (98.4, 1.6) ccw
  line L38 (-2, 1.6) -> (-2, -0.9)
  line L39 (-7, 4.1) -> (-4.5, 4.1)
  line L40 (100.9, 4.1) -> (98.4, 4.1)
  line L41 (95.9, -0.9) -> (95.9, 4.1)
  line L42 (95.9, -0.9) -> (98.4, -0.9)
  dimension "d412" = 5
  dimension "d414" = 0.8
  constraint coincident L0.start L5.end
  constraint perpendicular L5 L27
  constraint tangent L28 A20
  constraint tangent L29 A20
  constraint coincident L5 L30.end
  constraint tangent L30 A20
  constraint perpendicular L5 L30
  constraint concentric A17 A20
  constraint midpoint L32 L33.start
  constraint perpendicular L32 L33
  constraint symmetric L0.start L33 L36.start
  constraint symmetric L27.end L33 L34.start
  constraint symmetric L30.start L33 L35.start
  constraint symmetric L33 A19 A20
  constraint symmetric L28.end L33 L34.end
  constraint symmetric L29.end L33 L36.end
  constraint symmetric L30.end L33 L35.end
  constraint symmetric A17 L33 A18
  constraint perpendicular L34 L38
  measures "d412" distance of L0.start L27.end
  measures "d414" diameter of A17
extrude "Extrude45" add sketch "Sketch52" along normal blind 10.6 contours L0 L5 L27 L28 L29 L30 L31 A20 L40 L41 L42 | L34 L35 L36 L37 A19 L38 L39 bodies 3
sketch "Sketch53" plane through (0, 0, 10) normal (0, 0, -1) x (1, 0, 0)
  line L0 (46.4092, -77.2) -> (-2, -77.2)
  line L1 (-2, -77.2) -> (-2, -85.1)
  line L2 (-2, -85.1) -> (75.9, -85.1)
  line L3 (75.9, -85.1) -> (75.9, -77.2)
  line L4 (75.9, -77.2) -> (47.4908, -77.2)
  arc A0 (46.4092, -77.2) -> (47.4908, -77.2) centre (46.95, -80.1) ccw
  line L5 (-2, -81.15) -> (18, -81.15)
  circle A1 centre (8, -81.15) radius 2.5
  circle A2 centre (8, -81.15) radius 0.4
  line L6 (10.5, -81.15) -> (10.5, -77.2)
  line L7 (5.5, -81.15) -> (5.5, -77.2)
  line L8 (5.5, -77.2) -> (10.5, -77.2)
  line L9 (8, -81.15) -> (75.9, -81.15)
  line L10 (75.9, -81.15) -> (70.9, -81.15)
  circle A3 centre (73.4, -81.15) radius 2.5
  line L11 (70.9, -81.15) -> (70.9, -77.2)
  line L12 (75.9, -81.15) -> (75.9, -77.2)
  line L13 (75.9, -77.2) -> (70.9, -77.2)
  circle A4 centre (73.4, -81.15) radius 0.4
  dimension "d420" = 20
  dimension "d421" = 5
  dimension "d422" = 0.8
  dimension "d440" = 5
  dimension "d441" = 0.8
  constraint midpoint L1 L5.start
  constraint perpendicular L1 L5
  constraint midpoint L5 A1.centre
  constraint concentric A1 A2
  constraint coincident A1 L6.start
  constraint coincident L5 L6.start
  constraint coincident L0 L6.end
  constraint tangent A1 L6
  constraint coincident A1 L7.start
  constraint coincident L5 L7.start
  constraint coincident L0 L7.end
  constraint tangent A1 L7
  constraint coincident A1.centre A2.centre
  constraint midpoint L3 L9.end
  constraint perpendicular L3 L10
  constraint midpoint L10 A3.centre
  constraint coincident L10.end A3
  constraint tangent A3 L11
  constraint tangent A3 L12
  constraint coincident L3.end L4.start
  constraint coincident L4 L11.end
  constraint concentric A3 A4
  measures "d420" distance of L5.start L5.end
  measures "d421" diameter of A1
  measures "d422" diameter of A2
  measures "d440" distance of L9.end L10.end
  measures "d441" diameter of A4
extrude "Extrude46" add sketch "Sketch53" along normal blind 6 contours L0 A1 L6 L7 L8 | L5 A1 A2 L9 | L5 A1 A2 L9 | L9 L10 A3 A4 | L3 L4 A3 L11 L12 L13 | L9 L10 A3 A4 bodies 3
sketch "Sketch54" plane through (0, 0, -0.7) normal (0, 0, -1) x (1, 0, 0)
  circle A0 centre (10.06, -44.3) radius 2
  circle A1 centre (-14.9, 17.5) radius 2
  circle A2 centre (80.15, -44.4) radius 2
  circle A3 centre (103.9, 17.5) radius 2
  line L0 (77.6, 34.7) -> (16.3, 34.7)
  line L1 (16.3, 34.7) -> (16.3, 28.2)
  line L2 (16.3, 28.2) -> (18.6, 28.2)
  line L3 (18.6, 28.2) -> (18.6, 10.2)
  line L4 (18.6, 10.2) -> (16.3, 10.2)
  line L5 (16.3, 10.2) -> (16.3, 21)
  line L6 (16.3, 21) -> (-18.4, 21)
  line L7 (-18.4, 21) -> (-18.4, -42.54)
  line L8 (-18.4, -42.54) -> (6.28, -42.54)
  line L9 (6.28, -42.54) -> (6.28, -47.8)
  line L10 (6.28, -47.8) -> (69.9, -47.8)
  line L11 (69.9, -47.8) -> (69.9, -42)
  line L12 (69.9, -42) -> (76.4, -42)
  line L13 (76.4, -42) -> (76.4, -47.8)
  line L14 (76.4, -47.8) -> (83.9, -47.8)
  line L15 (83.9, -47.8) -> (83.9, -41.2)
  line L16 (83.9, -41.2) -> (95.4, -41.2)
  line L17 (95.4, -41.2) -> (95.4, -47.8)
  line L18 (95.4, -47.8) -> (107.4, -47.8)
  line L19 (107.4, -47.8) -> (107.4, 21)
  line L20 (107.4, 21) -> (77.6, 21)
  line L21 (77.6, 21) -> (77.6, 10.2)
  line L22 (77.6, 10.2) -> (75.3, 10.2)
  line L23 (75.3, 10.2) -> (75.3, 28.2)
  line L24 (75.3, 28.2) -> (77.6, 28.2)
  line L25 (77.6, 28.2) -> (77.6, 34.7)
  line L26 (107.4, -13.4) -> (84.4, -13.4)
  line L27 (84.4, -13.4) -> (84.4, 21)
  line L28 (84.4, 21) -> (84.4, -5)
  circle A4 centre (84.4, -5) radius 1.5
  line L29 (-18.4, -10.77) -> (-3.4, -10.77)
  line L30 (-3.4, -10.77) -> (-3.4, 21)
  line L31 (-3.4, 21) -> (-3.4, 0)
  circle A5 centre (-3.4, 0) radius 1.5
  dimension "d425" = 23
  dimension "d426" = 26
  dimension "d427" = 3
  dimension "d428" = 15
  dimension "d429" = 21
  dimension "d430" = 3
  constraint midpoint L19 L26.start
  constraint perpendicular L19 L26
  constraint coincident L20 L27.end
  constraint perpendicular L20 L27
  constraint perpendicular L20 L28
  constraint coincident L28.end A4.centre
  constraint midpoint L7 L29.start
  constraint perpendicular L7 L29
  constraint coincident L6 L30.end
  constraint perpendicular L6 L30
  constraint perpendicular L6 L31
  constraint coincident L31.end A5.centre
  measures "d425" distance of L26.start L26.end
  measures "d426" distance of L27.end L28.end
  measures "d427" diameter of A4
  measures "d428" distance of L29.start L29.end
  measures "d429" distance of L30.end L31.end
  measures "d430" diameter of A5
extrude "Extrude47" cut sketch "Sketch54" against normal blind 0.7 contours L27 L28 A4 | L27 L28 A4 | L30 L31 A5 | L30 L31 A5 bodies 2
move_body "Move20" bodies 2 to x (1, 0, 0) y (0, 1, 0) z (0, 0, 1) at (0, 0, 10)
sketch "Sketch55" plane through (0, 0, 4) normal (0, 0, -1) x (1, 0, 0)
  circle A0 centre (8, -81.15) radius 0.4
  circle A1 centre (-4.5, 1.6) radius 0.4
  circle A2 centre (98.4, 1.6) radius 0.4
  line L0 (95.9, 4.1) -> (93.9, 4.1)
  line L1 (93.9, 4.1) -> (93.9, -75.1)
  line L2 (93.9, -75.1) -> (0, -75.1)
  line L3 (0, -75.1) -> (0, 4.1)
  line L4 (0, 4.1) -> (-4.5, 4.1)
  line L5 (-4.5, 4.1) -> (-7, 4.1)
  line L6 (-7, 4.1) -> (-7, 1.6)
  arc A3 (-7, 1.6) -> (-4.5, -0.9) centre (-4.5, 1.6) ccw
  line L7 (-4.5, -0.9) -> (-2, -0.9)
  line L8 (-2, -0.9) -> (-2, -77.2)
  line L9 (-2, -77.2) -> (5.5, -77.2)
  line L10 (5.5, -77.2) -> (5.5, -81.15)
  arc A4 (5.5, -81.15) -> (10.5, -81.15) centre (8, -81.15) ccw
  line L11 (10.5, -81.15) -> (10.5, -77.2)
  line L12 (10.5, -77.2) -> (46.4092, -77.2)
  arc A5 (47.4908, -77.2) -> (46.4092, -77.2) centre (46.95, -80.1) ccw
  line L13 (47.4908, -77.2) -> (70.9, -77.2)
  line L14 (95.9, -77.2) -> (95.9, -0.9)
  line L15 (95.9, -0.9) -> (98.4, -0.9)
  arc A6 (98.4, -0.9) -> (100.9, 1.6) centre (98.4, 1.6) ccw
  line L16 (100.9, 1.6) -> (100.9, 4.1)
  line L17 (100.9, 4.1) -> (98.4, 4.1)
  line L18 (98.4, 4.1) -> (95.9, 4.1)
  line L19 (8, -81.15) -> (8, -83.65)
  line L20 (-2, -77.2) -> (-2, -85.1)
  line L21 (8, -83.65) -> (-2, -83.65)
  line L22 (-2, -83.65) -> (-2, -3.65)
  line L23 (-2, -3.65) -> (-7, -3.65)
  line L24 (-7, -3.65) -> (-7, 4.1)
  line L25 (-7, 4.1) -> (100.9, 4.1)
  line L26 (100.9, 4.1) -> (100.9, -3.65)
  line L27 (-2, -83.65) -> (70.9, -83.65)
  line L28 (95.9, -3.65) -> (100.9, -3.65)
  circle A7 centre (84.4, -5) radius 2.5
  circle A8 centre (84.4, -5) radius 1.5
  circle A9 centre (80.15, -44.4) radius 2.5
  circle A10 centre (80.15, -44.4) radius 2
  circle A11 centre (10.06, -44.3) radius 2
  line L29 (8.06, -44.3) -> (10.06, -44.3)
  circle A12 centre (98.4, 1.6) radius 1
  circle A13 centre (-4.5, 1.6) radius 1
  circle A14 centre (10.06, -44.3) radius 2.5
  circle A15 centre (8, -81.15) radius 1
  line L30 (70.9, -77.2) -> (70.9, -81.15)
  arc A16 (70.9, -81.15) -> (75.9, -81.15) centre (73.4, -81.15) ccw
  line L31 (75.9, -81.15) -> (75.9, -77.2)
  line L32 (75.9, -77.2) -> (95.9, -77.2)
  line L33 (75.9, -85.1) -> (75.9, -81.15)
  line L34 (70.9, -83.65) -> (75.9, -83.65)
  line L35 (75.9, -83.65) -> (95.9, -83.65)
  line L36 (95.9, -83.65) -> (95.9, -3.65)
  circle A17 centre (73.4, -81.15) radius 1
  point P0 (8.06, -44.3)
  dimension "d433" = 80
  dimension "d434" = 5
  dimension "d435" = 5
  dimension "d436" = 2
  dimension "d437" = 2
  dimension "d438" = 5
  dimension "d439" = 2
  dimension "d442" = 2
  constraint coincident A0.centre A4.centre
  constraint midpoint A4 L19.end
  constraint coincident L20 L21.end
  constraint tangent A4 L21
  constraint perpendicular L19 L21
  constraint coincident L8 L22.end
  constraint perpendicular L6 L23
  constraint coincident L5.end L6.start
  constraint perpendicular L23 L24
  constraint coincident L16.end L17.start
  constraint perpendicular L13 L26
  constraint perpendicular L19 L27
  constraint coincident L14 L28.start
  constraint concentric A7 A8
  constraint concentric A9 A10
  constraint coincident P0 L29.start
  constraint coincident A11.centre L29.end
  constraint concentric A2 A12
  constraint concentric A1 A13
  constraint concentric A0 A15
  constraint coincident L33 L34.end
  constraint perpendicular L14 L35
  constraint perpendicular L28 L36
  measures "d433" distance of L21.end L22.end
  measures "d434" diameter of A7
  measures "d435" diameter of A9
  measures "d436" diameter of A12
  measures "d437" diameter of A13
  measures "d438" diameter of A14
  measures "d439" diameter of A15
  measures "d442" diameter of A17
move_body "Move21" bodies 2 to x (1, 0, 0) y (0, 1, 0) z (0, 0, 1) at (0, 0, -20)
extrude "Extrude48" add sketch "Sketch55" along normal blind 1.6 separate body contours L0 L1 L2 L3 L4 L5 L6 A3 L7 L8 L9 L10 A4 L11 L12 A5 L13 L14 L15 A6 L16 L17 L18 L22 L24 L25 L26 L30 A16 L31 L32 L36 | L1 L2 L3 L25 | L14 L15 A6 L26 L28 | A3 L7 L8 L23 L24 | L31 L32 L33 L35 L36 | L9 L10 A4 L20 L21 L22 L27 | A16 L33 L34 | A4 L11 L12 A5 L13 L27 L30 A16 L34 makes body 8
sketch "Sketch57" plane through (-32.5, 0, 0) normal (-1, 0, 0) x (0, -1, 0)
  line L0 (25.3, 15.6) -> (-25.2, 15.6)
  line L1 (-25.2, 15.6) -> (-25.2, 14.6)
  line L2 (-25.2, 14.6) -> (4.1, 14.6)
  line L3 (4.1, 14.6) -> (4.1, 10)
  line L4 (4.1, 10) -> (25.3, 10)
  line L5 (25.3, 10) -> (25.3, 15.6)
  line L6 (35.3, 15.6) -> (25.3, 15.6)
  line L7 (35.3, 15.6) -> (32.8, 15.6)
  line L8 (35.3, 15.6) -> (35.3, 13.1)
  arc A0 (35.3, 13.1) -> (32.8, 15.6) centre (32.3361, 12.6361) ccw
  point P0 (35.3, 15.6)
  dimension "d449" = 2.5
  dimension "d450" = 2.5
  constraint coincident P0 L6.start
  constraint parallel L6 L7
  constraint perpendicular L6 L8
  measures "d449" distance of P0 L7.end
  measures "d450" distance of P0 L8.end
extrude "Extrude50" cut sketch "Sketch57" against normal blind 170 contours L6 L7 L8 A0 bodies 3
sketch "Sketch61" plane through (0, 0, 14.6) normal (0, 0, -1) x (1, 0, 0)
  circle A0 centre (117.6453, -56.4453) radius 2.85
  circle A1 centre (102.6547, -56.4453) radius 2.85
  line L0 (113.3329, -38.8299) -> (112.9477, -38.4448)
  line L1 (112.9477, -38.4448) -> (114.6448, -36.7477)
  line L2 (114.6448, -36.7477) -> (115.0299, -37.1329)
  arc A2 (122.2, -39.2591) -> (115.0299, -37.1329) centre (117.65, -41.45) ccw
  line L3 (122.2, -39.2591) -> (122.2, -43.6409)
  arc A3 (113.1, -43.6409) -> (122.2, -43.6409) centre (117.65, -41.45) ccw
  line L4 (113.1, -43.6409) -> (113.1, -39.2591)
  arc A4 (113.3329, -38.8299) -> (113.1, -39.2591) centre (117.65, -41.45) ccw
  line L5 (106.9671, -44.0701) -> (107.3523, -44.4552)
  line L6 (107.3523, -44.4552) -> (105.6552, -46.1523)
  line L7 (105.6552, -46.1523) -> (105.2701, -45.7671)
  arc A5 (98.115, -43.6717) -> (105.2701, -45.7671) centre (102.65, -41.45) ccw
  line L8 (98.115, -43.6717) -> (98.0852, -39.29)
  arc A6 (107.185, -39.2283) -> (98.0852, -39.29) centre (102.65, -41.45) ccw
  line L9 (107.185, -39.2283) -> (107.2148, -43.61)
  arc A7 (106.9671, -44.0701) -> (107.2148, -43.61) centre (102.65, -41.45) ccw
  line L10 (112.7701, -44.6329) -> (113.1552, -44.2477)
  line L11 (113.1552, -44.2477) -> (114.8523, -45.9448)
  line L12 (114.8523, -45.9448) -> (114.4671, -46.3299)
  arc A8 (112.3364, -53.5022) -> (114.4671, -46.3299) centre (110.15, -48.95) ccw
  line L13 (112.3364, -53.5022) -> (112.3364, -53.5)
  line L14 (112.3364, -53.5) -> (107.9591, -53.5)
  arc A9 (107.9591, -44.4) -> (107.9591, -53.5) centre (110.15, -48.95) ccw
  line L15 (107.9591, -44.4) -> (112.3409, -44.4)
  arc A10 (112.7701, -44.6329) -> (112.3409, -44.4) centre (110.15, -48.95) ccw
  line L16 (107.5299, -38.2671) -> (107.1448, -38.6523)
  line L17 (107.1448, -38.6523) -> (105.4477, -36.9552)
  line L18 (105.4477, -36.9552) -> (105.8329, -36.5701)
  arc A11 (107.9591, -29.4) -> (105.8329, -36.5701) centre (110.15, -33.95) ccw
  line L19 (107.9591, -29.4) -> (112.3409, -29.4)
  arc A12 (112.3409, -38.5) -> (112.3409, -29.4) centre (110.15, -33.95) ccw
  line L20 (112.3409, -38.5) -> (107.9591, -38.5)
  arc A13 (107.5299, -38.2671) -> (107.9591, -38.5) centre (110.15, -33.95) ccw
  line L21 (100.9, 4.1) -> (100.9, 1.6)
  arc A14 (98.4, -0.9) -> (100.9, 1.6) centre (98.4, 1.6) ccw
  line L22 (98.4, -0.9) -> (95.9, -0.9)
  line L23 (95.9, -0.9) -> (95.9, -77.2)
  line L24 (95.9, -77.2) -> (75.9, -77.2)
  line L25 (75.9, -77.2) -> (75.9, -85.1)
  line L26 (75.9, -85.1) -> (106.4, -85.1)
  arc A15 (106.4, -85.1) -> (126.4, -65.1) centre (106.4, -65.1) ccw
  line L27 (126.4, -65.1) -> (126.4, 4.1)
  line L28 (126.4, 4.1) -> (100.9, 4.1)
  circle A16 centre (110.15, -62.1) radius 2.5
  circle A17 centre (110.2363, -20.8316) radius 2.5
  line L29 (110.15, -48.95) -> (110.15, -33.95)
  line L30 (102.65, -41.45) -> (117.65, -41.45)
  line L31 (110.15, -41.45) -> (110.15, -43.95)
  line L32 (110.15, -43.95) -> (112.65, -43.95)
  line L33 (110.15, -41.45) -> (110.15, -38.95)
  line L34 (110.15, -38.95) -> (107.65, -38.95)
  line L35 (112.65, -43.95) -> (107.65, -43.95)
  line L36 (107.65, -43.95) -> (107.65, -38.95)
  line L37 (107.65, -38.95) -> (112.65, -38.95)
  line L38 (112.65, -38.95) -> (112.65, -43.95)
  dimension "d453" = 2.5
  dimension "d454" = 2.5
  dimension "d455" = 2.5
  dimension "d456" = 2.5
  constraint coincident A8.centre A9.centre
  constraint coincident A11.centre A12.centre
  constraint coincident A5.centre A6.centre
  constraint coincident A2.centre A3.centre
  constraint midpoint L29 L31.start
  constraint perpendicular L15 L31
  constraint perpendicular L31 L32
  constraint perpendicular L30 L33
  constraint perpendicular L29 L34
  constraint horizontal L35
  constraint vertical L36
  constraint horizontal L37
  constraint vertical L38
  measures "d453" distance of L31.start L31.end
  measures "d454" distance of L31.end L32.end
  measures "d455" distance of L31.start L33.end
  measures "d456" distance of L33.end L34.end
extrude "Extrude51" cut sketch "Sketch61" against normal blind 0.5 contours L29 L30 L31 L35 L36 | L29 L30 L31 L32 L35 L38 | L29 L30 L33 L34 L36 L37 | L29 L30 L33 L37 L38 bodies 3
move_body "Move22" bodies 2 to x (1, 0, 0) y (0, 1, 0) z (0, 0, 1) at (0, 0, 5)